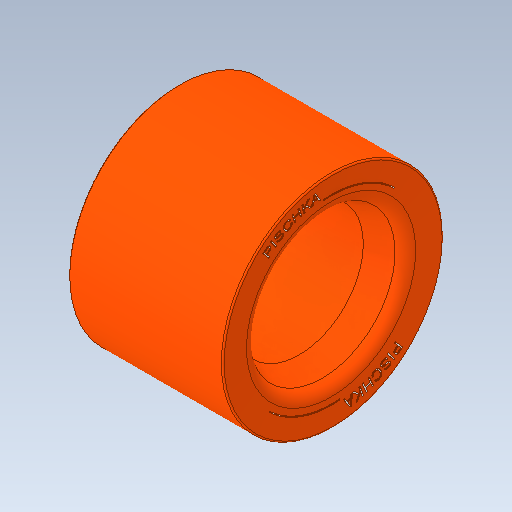
# Autodesk Inventor part: Kegel_urethane
Saved by Autodesk Inventor 2020.1 (Build 241239000, 239)
## iProperties
Created: 2018-01-15
Part Number: Kegel_urethane
Material: Rubber, Silicone
Document SubType Name: Modeling
Designer: Tobias
Density: 1.25 g/cm^3
Appearance: Rubber - Orangatang
Mass: 215.394 g
Surface Area: 276.313 cm^2
Volume: 172.315 cm^3
Author: Tobias
Autodesk Inventor part; units mm, degrees
ref_plane "YZ Plane" through (0, 0, 0) normal (1, 0, 0) x (0, 1, 0)
ref_plane "XZ Plane" through (0, 0, 0) normal (0, 1, 0) x (-1, 0, 0)
sketch "Sketch1" plane through (0, 0, 0) normal (0, 0, 1) x (1, 0, 0)
  line L0 (-35.8, 0) -> (42.6, 0) projected
  line L1 (30.3064, 27.5) -> (19, 23.25)
  line L2 (19, 23.25) -> (-19, 23.25)
  line L3 (-24.1407, 34.75) -> (-23.2, 34.75)
  line L4 (-23.2, 34.75) -> (-23.2, 31.5)
  line L5 (-23.2, 31.5) -> (-19, 31.5)
  line L6 (-19, 31.5) -> (-19, 23.25)
  line L7 (31.4, 40) -> (30.3064, 27.5)
  line L8 (-24.6, 40) -> (-24.1407, 34.75)
  line L9 (-24.6, 40) -> (31.4, 40)
  line L10 (0, 48) -> (0, -8) projected
  point P0 (0, 0)
  dimension "d27" = 46.5
  dimension "d29" = 69.5
  dimension "d31" = 63
  dimension "d35" = 55
  dimension "d39" = 80
  dimension "d40" = 1.4
  dimension "d42" = 5.6
  dimension "d44" = 19
  dimension "d45" = 19
  dimension "d46" = 56
  dimension "d47" = 5
  dimension "d48" = 5
  dimension "d49" = 12.5
  constraints: 18 end point, 3 perpendicular, 2 horizontal
  measures "d27" diameter of L2 L0
  measures "d29" diameter of L3 L0
  measures "d31" diameter of L5 L0
  measures "d35" diameter of L1.start L0
  measures "d39" diameter of L9 L0
  measures "d40" distance from line of L8.start L4
  measures "d42" distance from line of L6 L8.start
  measures "d44" distance between parallel lines of L10 L6
  measures "d45" distance from line of L10 L1.end
  measures "d46" distance of L8.start L7.start
  measures "d47" angle of L10 L8
  measures "d48" angle of L10 L7
  measures "d49" distance from line of L1.start L9
revolve "Revolution1" add sketch "Sketch1" angle 360 about axis through (0, 0, 0) along (1, 0, 0)
fillet "Fillet8" radius 7 1 edges at (-19, -31.5, 0)
fillet "Fillet9" radius 7 1 edges at (-23.2, -31.5, 0)
fillet "Fillet10" radius 6 1 edges at (-23.2, -34.75, 0)
fillet "Fillet11" radius 5 1 edges at (30.3064, -27.5, 0)
fillet "Fillet12" radius 0.5 2 edges at (31.4, -40, 0) (-24.6, -40, 0)
ref_plane "Work Plane2" through (31.4, 40, 0) normal (1, 0, 0) x (0, 1, 0)
sketch "Sketch4" plane through (31.4, 40, 0) normal (1, 0, 0) x (0, 1, 0)
  circle A0 centre (-40, 0) radius 30.6366 construction
  line L0 (-64.5965, -22.9785) -> (-67.2414, -25.2708)
  line L1 (-67.2414, -25.2708) -> (-68.1062, -24.2729)
  spline S0 degree 2 poles (-68.1062, -24.2729) (-68.3351, -24.0088) (-68.4295, -23.847) knots 0 0 0 1 1 1
  spline S1 degree 2 poles (-68.4295, -23.847) (-68.5667, -23.6235) (-68.6124, -23.2042) (-68.4236, -22.7581) (-68.226, -22.5869) knots 0 0 0 1 2 3 3 3
  spline S2 degree 2 poles (-68.226, -22.5869) (-67.8893, -22.2951) (-67.0495, -22.3192) (-66.5638, -22.8796) knots 0 0 0 1 2 2 2
  line L2 (-66.5638, -22.8796) -> (-65.975, -23.559)
  line L3 (-65.975, -23.559) -> (-64.9005, -22.6277)
  line L4 (-64.9005, -22.6277) -> (-64.5965, -22.9785)
  line L5 (-66.2875, -23.8298) -> (-66.8798, -23.1464)
  spline S3 degree 2 poles (-66.8798, -23.1464) (-67.175, -22.8057) (-67.6734, -22.7398) (-67.9032, -22.939) knots 0 0 0 1 2 2 2
  spline S4 degree 2 poles (-67.9032, -22.939) (-68.0685, -23.0823) (-68.1613, -23.4558) (-68.0788, -23.6243) knots 0 0 0 1 2 2 2
  spline S5 degree 2 poles (-68.0788, -23.6243) (-68.0261, -23.734) (-67.82, -23.9718) knots 0 0 0 1 1 1
  line L6 (-67.82, -23.9718) -> (-67.2329, -24.6492)
  line L7 (-67.2329, -24.6492) -> (-66.2875, -23.8298)
  line L8 (-66.7357, -20.4127) -> (-69.5315, -22.5182)
  line L9 (-69.5315, -22.5182) -> (-69.8108, -22.1474)
  line L10 (-69.8108, -22.1474) -> (-67.0149, -20.0419)
  line L11 (-67.0149, -20.0419) -> (-66.7357, -20.4127)
  line L12 (-68.3675, -20.1421) -> (-68.6374, -19.7958)
  spline S6 degree 2 poles (-68.6374, -19.7958) (-68.4335, -19.6249) (-68.2754, -19.2515) (-68.3614, -18.7378) (-68.5244, -18.4874) knots 0 0 0 1 2 3 3 3
  spline S7 degree 2 poles (-68.5244, -18.4874) (-68.6684, -18.266) (-69.0229, -18.0097) (-69.3609, -17.9941) (-69.4973, -18.0828) knots 0 0 0 1 2 3 3 3
  spline S8 degree 2 poles (-69.4973, -18.0828) (-69.6359, -18.173) (-69.7383, -18.4656) (-69.6869, -18.6963) knots 0 0 0 1 2 2 2
  spline S9 degree 2 poles (-69.6869, -18.6963) (-69.6567, -18.8454) (-69.3232, -19.7837) (-69.3042, -20.0036) knots 0 0 0 1 2 2 2
  spline S10 degree 2 poles (-69.3042, -20.0036) (-69.277, -20.2851) (-69.4696, -20.7032) (-69.6708, -20.8342) knots 0 0 0 1 2 2 2
  spline S11 degree 2 poles (-69.6708, -20.8342) (-69.8944, -20.9797) (-70.4434, -20.9772) (-70.9604, -20.6229) (-71.1539, -20.3255) knots 0 0 0 1 2 3 3 3
  spline S12 degree 2 poles (-71.1539, -20.3255) (-71.3663, -19.9991) (-71.4805, -19.3637) (-71.2474, -18.8269) (-70.9961, -18.6506) knots 0 0 0 1 2 3 3 3
  line L13 (-70.9961, -18.6506) -> (-70.7255, -19.0029)
  spline S13 degree 2 poles (-70.7255, -19.0029) (-70.9861, -19.2138) (-71.0431, -19.7474) (-70.822, -20.0873) knots 0 0 0 1 2 2 2
  spline S14 degree 2 poles (-70.822, -20.0873) (-70.5921, -20.4406) (-70.1218, -20.5961) (-69.9406, -20.4782) knots 0 0 0 1 2 2 2
  spline S15 degree 2 poles (-69.9406, -20.4782) (-69.7819, -20.3749) (-69.7532, -20.194) knots 0 0 0 1 1 1
  spline S16 degree 2 poles (-69.7532, -20.194) (-69.7268, -20.0144) (-70.1304, -18.9245) (-70.1649, -18.6954) knots 0 0 0 1 2 2 2
  spline S17 degree 2 poles (-70.1649, -18.6954) (-70.2122, -18.3634) (-70.0086, -17.884) (-69.7738, -17.7312) knots 0 0 0 1 2 2 2
  spline S18 degree 2 poles (-69.7738, -17.7312) (-69.539, -17.5785) (-68.9507, -17.5777) (-68.3931, -17.9309) (-68.1894, -18.244) knots 0 0 0 1 2 3 3 3
  spline S19 degree 2 poles (-68.1894, -18.244) (-67.929, -18.6442) (-67.8124, -19.3322) (-68.0781, -19.9411) (-68.3675, -20.1421) knots 0 0 0 1 2 3 3 3
  line L14 (-71.4992, -14.9899) -> (-71.6075, -14.5235)
  spline S20 degree 2 poles (-71.6075, -14.5235) (-71.0328, -14.3924) (-70.1534, -14.7884) (-69.9029, -15.2745) knots 0 0 0 1 2 2 2
  spline S21 degree 2 poles (-69.9029, -15.2745) (-69.6438, -15.7772) (-69.7289, -16.6194) (-70.3344, -17.3487) (-70.7802, -17.5785) knots 0 0 0 1 2 3 3 3
  spline S22 degree 2 poles (-70.7802, -17.5785) (-71.2663, -17.829) (-72.1838, -17.8307) (-72.9117, -17.3385) (-73.1243, -16.9259) knots 0 0 0 1 2 3 3 3
  spline S23 degree 2 poles (-73.1243, -16.9259) (-73.3651, -16.4588) (-73.216, -15.5776) (-72.8516, -15.2307) knots 0 0 0 1 2 2 2
  line L15 (-72.8516, -15.2307) -> (-72.5454, -15.5861)
  spline S24 degree 2 poles (-72.5454, -15.5861) (-72.8282, -15.87) (-72.9274, -16.4403) (-72.7661, -16.7533) knots 0 0 0 1 2 2 2
  spline S25 degree 2 poles (-72.7661, -16.7533) (-72.5816, -17.1114) (-71.9884, -17.4179) (-71.3096, -17.3141) (-71.0013, -17.1552) knots 0 0 0 1 2 3 3 3
  spline S26 degree 2 poles (-71.0013, -17.1552) (-70.6053, -16.9511) (-70.1323, -16.4132) (-70.0912, -15.7768) (-70.2379, -15.4922) knots 0 0 0 1 2 3 3 3
  spline S27 degree 2 poles (-70.2379, -15.4922) (-70.4163, -15.146) (-71.0615, -14.8723) (-71.4992, -14.9899) knots 0 0 0 1 2 2 2
  line L16 (-70.8511, -13.4728) -> (-74.1129, -14.7417)
  line L17 (-74.1129, -14.7417) -> (-74.2812, -14.3091)
  line L18 (-74.2812, -14.3091) -> (-72.9412, -13.7878)
  line L19 (-72.9412, -13.7878) -> (-73.5988, -12.0972)
  line L20 (-73.5988, -12.0972) -> (-74.9389, -12.6185)
  line L21 (-74.9389, -12.6185) -> (-75.1072, -12.1859)
  line L22 (-75.1072, -12.1859) -> (-71.8453, -10.917)
  line L23 (-71.8453, -10.917) -> (-71.677, -11.3496)
  line L24 (-71.677, -11.3496) -> (-73.2135, -11.9473)
  line L25 (-73.2135, -11.9473) -> (-72.5558, -13.6379)
  line L26 (-72.5558, -13.6379) -> (-71.0193, -13.0402)
  line L27 (-71.0193, -13.0402) -> (-70.8511, -13.4728)
  line L28 (-72.0774, -10.2024) -> (-75.4505, -11.1362)
  line L29 (-75.4505, -11.1362) -> (-75.5743, -10.6889)
  line L30 (-75.5743, -10.6889) -> (-73.9032, -10.2262)
  line L31 (-73.9032, -10.2262) -> (-76.0384, -9.0126)
  line L32 (-76.0384, -9.0126) -> (-76.2057, -8.4084)
  line L33 (-76.2057, -8.4084) -> (-74.4464, -9.4438)
  line L34 (-74.4464, -9.4438) -> (-72.8496, -7.4129)
  line L35 (-72.8496, -7.4129) -> (-72.6866, -8.0016)
  line L36 (-72.6866, -8.0016) -> (-74.0588, -9.6742)
  line L37 (-74.0588, -9.6742) -> (-73.371, -10.0789)
  line L38 (-73.371, -10.0789) -> (-72.2012, -9.755)
  line L39 (-72.2012, -9.755) -> (-72.0774, -10.2024)
  line L40 (-72.8519, -7.4079) -> (-76.5311, -6.6858)
  line L41 (-76.5311, -6.6858) -> (-76.6174, -6.1918)
  line L42 (-76.6174, -6.1918) -> (-73.4157, -4.1809)
  line L43 (-73.4157, -4.1809) -> (-73.3248, -4.7012)
  line L44 (-73.3248, -4.7012) -> (-74.2983, -5.2829)
  line L45 (-74.2983, -5.2829) -> (-74.0457, -6.7282)
  line L46 (-74.0457, -6.7282) -> (-72.9364, -6.9244)
  line L47 (-72.9364, -6.9244) -> (-72.8519, -7.4079)
  line L48 (-74.4392, -6.6616) -> (-74.644, -5.4896)
  line L49 (-74.644, -5.4896) -> (-75.5372, -6.0193)
  spline S28 degree 2 poles (-75.5372, -6.0193) (-75.9449, -6.2585) (-76.2097, -6.386) knots 0 0 0 1 1 1
  spline S29 degree 2 poles (-76.2097, -6.386) (-75.8667, -6.3965) (-75.5175, -6.4573) knots 0 0 0 1 1 1
  line L50 (-75.5175, -6.4573) -> (-74.4392, -6.6616)
  line L51 (-72.5749, -2.8572) -> (-72.8841, -2.8701)
  line L52 (-72.8841, -2.8701) -> (-73.0027, -0.0235)
  line L53 (-73.0027, -0.0235) -> (-72.6935, -0.0106)
  line L54 (-72.6935, -0.0106) -> (-72.5749, -2.8572)
  line L55 (-72.6998, -0.0928) -> (-73.009, -0.0795)
  line L56 (-73.009, -0.0795) -> (-72.8865, 2.767)
  line L57 (-72.8865, 2.767) -> (-72.5773, 2.7537)
  line L58 (-72.5773, 2.7537) -> (-72.6998, -0.0928)
  line L59 (-72.5906, 2.6723) -> (-72.8975, 2.7117)
  line L60 (-72.8975, 2.7117) -> (-72.5348, 5.5376)
  line L61 (-72.5348, 5.5376) -> (-72.2278, 5.4982)
  line L62 (-72.2278, 5.4982) -> (-72.5906, 2.6723)
  line L63 (-72.248, 5.4183) -> (-72.5505, 5.4835)
  line L64 (-72.5505, 5.4835) -> (-71.95, 8.2686)
  line L65 (-71.95, 8.2686) -> (-71.6475, 8.2034)
  line L66 (-71.6475, 8.2034) -> (-72.248, 5.4183)
  line L67 (-71.6744, 8.1255) -> (-71.9703, 8.216)
  line L68 (-71.9703, 8.216) -> (-71.1365, 10.9404)
  line L69 (-71.1365, 10.9404) -> (-70.8406, 10.8498)
  line L70 (-70.8406, 10.8498) -> (-71.6744, 8.1255)
  line L71 (-70.8739, 10.7745) -> (-71.1611, 10.8897)
  line L72 (-71.1611, 10.8897) -> (-70.1, 13.5338)
  line L73 (-70.1, 13.5338) -> (-69.8128, 13.4186)
  line L74 (-69.8128, 13.4186) -> (-70.8739, 10.7745)
  line L75 (-69.8524, 13.3463) -> (-70.1288, 13.4854)
  line L76 (-70.1288, 13.4854) -> (-68.848, 16.0303)
  line L77 (-68.848, 16.0303) -> (-68.5715, 15.8912)
  line L78 (-68.5715, 15.8912) -> (-69.8524, 13.3463)
  line L79 (-68.6171, 15.8225) -> (-68.8807, 15.9845)
  line L80 (-68.8807, 15.9845) -> (-67.3893, 18.412)
  line L81 (-67.3893, 18.412) -> (-67.1256, 18.25)
  line L82 (-67.1256, 18.25) -> (-68.6171, 15.8225)
  line L83 (-67.1768, 18.1854) -> (-67.4258, 18.3691)
  line L84 (-67.4258, 18.3691) -> (-65.7345, 20.6619)
  line L85 (-65.7345, 20.6619) -> (-65.4854, 20.4782)
  line L86 (-65.4854, 20.4782) -> (-67.1768, 18.1854)
  line L87 (-65.5419, 20.4181) -> (-65.7745, 20.6222)
  line L88 (-65.7745, 20.6222) -> (-63.8954, 22.7637)
  line L89 (-63.8954, 22.7637) -> (-63.6628, 22.5596)
  line L90 (-63.6628, 22.5596) -> (-65.5419, 20.4181)
  line L91 (-15.4035, 22.9785) -> (-12.7586, 25.2708)
  line L92 (-12.7586, 25.2708) -> (-11.8938, 24.2729)
  spline S30 degree 2 poles (-11.8938, 24.2729) (-11.6649, 24.0088) (-11.5705, 23.847) knots 0 0 0 1 1 1
  spline S31 degree 2 poles (-11.5705, 23.847) (-11.4333, 23.6235) (-11.3876, 23.2042) (-11.5764, 22.7581) (-11.774, 22.5869) knots 0 0 0 1 2 3 3 3
  spline S32 degree 2 poles (-11.774, 22.5869) (-12.1107, 22.2951) (-12.9505, 22.3192) (-13.4362, 22.8796) knots 0 0 0 1 2 2 2
  line L93 (-13.4362, 22.8796) -> (-14.025, 23.559)
  line L94 (-14.025, 23.559) -> (-15.0995, 22.6277)
  line L95 (-15.0995, 22.6277) -> (-15.4035, 22.9785)
  line L96 (-13.7125, 23.8298) -> (-13.1202, 23.1464)
  spline S33 degree 2 poles (-13.1202, 23.1464) (-12.825, 22.8057) (-12.3266, 22.7398) (-12.0968, 22.939) knots 0 0 0 1 2 2 2
  spline S34 degree 2 poles (-12.0968, 22.939) (-11.9315, 23.0823) (-11.8387, 23.4558) (-11.9212, 23.6243) knots 0 0 0 1 2 2 2
  spline S35 degree 2 poles (-11.9212, 23.6243) (-11.9739, 23.734) (-12.18, 23.9718) knots 0 0 0 1 1 1
  line L97 (-12.18, 23.9718) -> (-12.7671, 24.6492)
  line L98 (-12.7671, 24.6492) -> (-13.7125, 23.8298)
  line L99 (-13.2643, 20.4127) -> (-10.4685, 22.5182)
  line L100 (-10.4685, 22.5182) -> (-10.1892, 22.1474)
  line L101 (-10.1892, 22.1474) -> (-12.9851, 20.0419)
  line L102 (-12.9851, 20.0419) -> (-13.2643, 20.4127)
  line L103 (-11.6325, 20.1421) -> (-11.3626, 19.7958)
  spline S36 degree 2 poles (-11.3626, 19.7958) (-11.5665, 19.6249) (-11.7246, 19.2515) (-11.6386, 18.7378) (-11.4756, 18.4874) knots 0 0 0 1 2 3 3 3
  spline S37 degree 2 poles (-11.4756, 18.4874) (-11.3316, 18.266) (-10.9771, 18.0097) (-10.6391, 17.9941) (-10.5027, 18.0828) knots 0 0 0 1 2 3 3 3
  spline S38 degree 2 poles (-10.5027, 18.0828) (-10.3641, 18.173) (-10.2617, 18.4656) (-10.3131, 18.6963) knots 0 0 0 1 2 2 2
  spline S39 degree 2 poles (-10.3131, 18.6963) (-10.3433, 18.8454) (-10.6768, 19.7837) (-10.6958, 20.0036) knots 0 0 0 1 2 2 2
  spline S40 degree 2 poles (-10.6958, 20.0036) (-10.723, 20.2851) (-10.5304, 20.7032) (-10.3292, 20.8342) knots 0 0 0 1 2 2 2
  spline S41 degree 2 poles (-10.3292, 20.8342) (-10.1056, 20.9797) (-9.5566, 20.9772) (-9.0396, 20.6229) (-8.8461, 20.3255) knots 0 0 0 1 2 3 3 3
  spline S42 degree 2 poles (-8.8461, 20.3255) (-8.6337, 19.9991) (-8.5195, 19.3637) (-8.7526, 18.8269) (-9.0039, 18.6506) knots 0 0 0 1 2 3 3 3
  line L104 (-9.0039, 18.6506) -> (-9.2745, 19.0029)
  spline S43 degree 2 poles (-9.2745, 19.0029) (-9.0139, 19.2138) (-8.9569, 19.7474) (-9.178, 20.0873) knots 0 0 0 1 2 2 2
  spline S44 degree 2 poles (-9.178, 20.0873) (-9.4079, 20.4406) (-9.8782, 20.5961) (-10.0594, 20.4782) knots 0 0 0 1 2 2 2
  spline S45 degree 2 poles (-10.0594, 20.4782) (-10.2181, 20.3749) (-10.2468, 20.194) knots 0 0 0 1 1 1
  spline S46 degree 2 poles (-10.2468, 20.194) (-10.2732, 20.0144) (-9.8696, 18.9245) (-9.8351, 18.6954) knots 0 0 0 1 2 2 2
  spline S47 degree 2 poles (-9.8351, 18.6954) (-9.7878, 18.3634) (-9.9914, 17.884) (-10.2262, 17.7312) knots 0 0 0 1 2 2 2
  spline S48 degree 2 poles (-10.2262, 17.7312) (-10.461, 17.5785) (-11.0493, 17.5777) (-11.6069, 17.9309) (-11.8106, 18.244) knots 0 0 0 1 2 3 3 3
  spline S49 degree 2 poles (-11.8106, 18.244) (-12.071, 18.6442) (-12.1876, 19.3322) (-11.9219, 19.9411) (-11.6325, 20.1421) knots 0 0 0 1 2 3 3 3
  line L105 (-8.5008, 14.9899) -> (-8.3925, 14.5235)
  spline S50 degree 2 poles (-8.3925, 14.5235) (-8.9672, 14.3924) (-9.8466, 14.7884) (-10.0971, 15.2745) knots 0 0 0 1 2 2 2
  spline S51 degree 2 poles (-10.0971, 15.2745) (-10.3562, 15.7772) (-10.2711, 16.6194) (-9.6656, 17.3487) (-9.2198, 17.5785) knots 0 0 0 1 2 3 3 3
  spline S52 degree 2 poles (-9.2198, 17.5785) (-8.7337, 17.829) (-7.8162, 17.8307) (-7.0883, 17.3385) (-6.8757, 16.9259) knots 0 0 0 1 2 3 3 3
  spline S53 degree 2 poles (-6.8757, 16.9259) (-6.6349, 16.4588) (-6.784, 15.5776) (-7.1484, 15.2307) knots 0 0 0 1 2 2 2
  line L106 (-7.1484, 15.2307) -> (-7.4546, 15.5861)
  spline S54 degree 2 poles (-7.4546, 15.5861) (-7.1718, 15.87) (-7.0726, 16.4403) (-7.2339, 16.7533) knots 0 0 0 1 2 2 2
  spline S55 degree 2 poles (-7.2339, 16.7533) (-7.4184, 17.1114) (-8.0116, 17.4179) (-8.6904, 17.3141) (-8.9987, 17.1552) knots 0 0 0 1 2 3 3 3
  spline S56 degree 2 poles (-8.9987, 17.1552) (-9.3947, 16.9511) (-9.8677, 16.4132) (-9.9088, 15.7768) (-9.7621, 15.4922) knots 0 0 0 1 2 3 3 3
  spline S57 degree 2 poles (-9.7621, 15.4922) (-9.5837, 15.146) (-8.9385, 14.8723) (-8.5008, 14.9899) knots 0 0 0 1 2 2 2
  line L107 (-9.1489, 13.4728) -> (-5.8871, 14.7417)
  line L108 (-5.8871, 14.7417) -> (-5.7188, 14.3091)
  line L109 (-5.7188, 14.3091) -> (-7.0588, 13.7878)
  line L110 (-7.0588, 13.7878) -> (-6.4012, 12.0972)
  line L111 (-6.4012, 12.0972) -> (-5.0611, 12.6185)
  line L112 (-5.0611, 12.6185) -> (-4.8928, 12.1859)
  line L113 (-4.8928, 12.1859) -> (-8.1547, 10.917)
  line L114 (-8.1547, 10.917) -> (-8.323, 11.3496)
  line L115 (-8.323, 11.3496) -> (-6.7865, 11.9473)
  line L116 (-6.7865, 11.9473) -> (-7.4442, 13.6379)
  line L117 (-7.4442, 13.6379) -> (-8.9807, 13.0402)
  line L118 (-8.9807, 13.0402) -> (-9.1489, 13.4728)
  line L119 (-7.9226, 10.2024) -> (-4.5495, 11.1362)
  line L120 (-4.5495, 11.1362) -> (-4.4257, 10.6889)
  line L121 (-4.4257, 10.6889) -> (-6.0968, 10.2262)
  line L122 (-6.0968, 10.2262) -> (-3.9616, 9.0126)
  line L123 (-3.9616, 9.0126) -> (-3.7943, 8.4084)
  line L124 (-3.7943, 8.4084) -> (-5.5536, 9.4438)
  line L125 (-5.5536, 9.4438) -> (-7.1504, 7.4129)
  line L126 (-7.1504, 7.4129) -> (-7.3134, 8.0016)
  line L127 (-7.3134, 8.0016) -> (-5.9412, 9.6742)
  line L128 (-5.9412, 9.6742) -> (-6.629, 10.0789)
  line L129 (-6.629, 10.0789) -> (-7.7988, 9.755)
  line L130 (-7.7988, 9.755) -> (-7.9226, 10.2024)
  line L131 (-7.1481, 7.4079) -> (-3.4689, 6.6858)
  line L132 (-3.4689, 6.6858) -> (-3.3826, 6.1918)
  line L133 (-3.3826, 6.1918) -> (-6.5843, 4.1809)
  line L134 (-6.5843, 4.1809) -> (-6.6752, 4.7012)
  line L135 (-6.6752, 4.7012) -> (-5.7017, 5.2829)
  line L136 (-5.7017, 5.2829) -> (-5.9543, 6.7282)
  line L137 (-5.9543, 6.7282) -> (-7.0636, 6.9244)
  line L138 (-7.0636, 6.9244) -> (-7.1481, 7.4079)
  line L139 (-5.5608, 6.6616) -> (-5.356, 5.4896)
  line L140 (-5.356, 5.4896) -> (-4.4628, 6.0193)
  spline S58 degree 2 poles (-4.4628, 6.0193) (-4.0551, 6.2585) (-3.7903, 6.386) knots 0 0 0 1 1 1
  spline S59 degree 2 poles (-3.7903, 6.386) (-4.1333, 6.3965) (-4.4825, 6.4573) knots 0 0 0 1 1 1
  line L141 (-4.4825, 6.4573) -> (-5.5608, 6.6616)
  line L142 (-7.4251, 2.8572) -> (-7.1159, 2.8701)
  line L143 (-7.1159, 2.8701) -> (-6.9973, 0.0235)
  line L144 (-6.9973, 0.0235) -> (-7.3065, 0.0106)
  line L145 (-7.3065, 0.0106) -> (-7.4251, 2.8572)
  line L146 (-7.3002, 0.0928) -> (-6.991, 0.0795)
  line L147 (-6.991, 0.0795) -> (-7.1135, -2.767)
  line L148 (-7.1135, -2.767) -> (-7.4227, -2.7537)
  line L149 (-7.4227, -2.7537) -> (-7.3002, 0.0928)
  line L150 (-7.4094, -2.6723) -> (-7.1025, -2.7117)
  line L151 (-7.1025, -2.7117) -> (-7.4652, -5.5376)
  line L152 (-7.4652, -5.5376) -> (-7.7722, -5.4982)
  line L153 (-7.7722, -5.4982) -> (-7.4094, -2.6723)
  line L154 (-7.752, -5.4183) -> (-7.4495, -5.4835)
  line L155 (-7.4495, -5.4835) -> (-8.05, -8.2686)
  line L156 (-8.05, -8.2686) -> (-8.3525, -8.2034)
  line L157 (-8.3525, -8.2034) -> (-7.752, -5.4183)
  line L158 (-8.3256, -8.1255) -> (-8.0297, -8.216)
  line L159 (-8.0297, -8.216) -> (-8.8635, -10.9404)
  line L160 (-8.8635, -10.9404) -> (-9.1594, -10.8498)
  line L161 (-9.1594, -10.8498) -> (-8.3256, -8.1255)
  line L162 (-9.1261, -10.7745) -> (-8.8389, -10.8897)
  line L163 (-8.8389, -10.8897) -> (-9.9, -13.5338)
  line L164 (-9.9, -13.5338) -> (-10.1872, -13.4186)
  line L165 (-10.1872, -13.4186) -> (-9.1261, -10.7745)
  line L166 (-10.1476, -13.3463) -> (-9.8712, -13.4854)
  line L167 (-9.8712, -13.4854) -> (-11.152, -16.0303)
  line L168 (-11.152, -16.0303) -> (-11.4285, -15.8912)
  line L169 (-11.4285, -15.8912) -> (-10.1476, -13.3463)
  line L170 (-11.3829, -15.8225) -> (-11.1193, -15.9845)
  line L171 (-11.1193, -15.9845) -> (-12.6107, -18.412)
  line L172 (-12.6107, -18.412) -> (-12.8744, -18.25)
  line L173 (-12.8744, -18.25) -> (-11.3829, -15.8225)
  line L174 (-12.8232, -18.1854) -> (-12.5742, -18.3691)
  line L175 (-12.5742, -18.3691) -> (-14.2655, -20.6619)
  line L176 (-14.2655, -20.6619) -> (-14.5146, -20.4782)
  line L177 (-14.5146, -20.4782) -> (-12.8232, -18.1854)
  line L178 (-14.4581, -20.4181) -> (-14.2255, -20.6222)
  line L179 (-14.2255, -20.6222) -> (-16.1046, -22.7637)
  line L180 (-16.1046, -22.7637) -> (-16.3372, -22.5596)
  line L181 (-16.3372, -22.5596) -> (-14.4581, -20.4181)
  point P0 (-40, 0)
  constraints: 1 centre point, 2 other
emboss "Emboss1" sketch "Sketch4" operation add depth 0.1 direction (-1, 0, 0)
body "Solid1"
